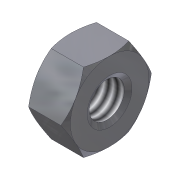
# Autodesk Inventor part: ANSI B18.2.2 - 1/4 - 20
Saved by Autodesk Inventor 2012 SP1 (Build 160190100, 190)
## iProperties
Library Location: D:\Program Files\Autodesk\Inventor 6\content
Library: local
SubLibrary: ANSI
Family: 1001
Member: 10
Member Major Revision: 1
Member Minor Revision: 2
Comments: To add or edit properties for Autodesk Inventor files, use iProperties.
Created: 2003-01-12
Part Number: ANSI B18.2.2 - 1/4 - 20
Vendor: Autodesk Inc.
Document SubType Name: Modeling
Designer: geyerm
Description: Hex Nut
Standard: ANSI B18.2.2 1/4 - 20
Material: Steel, High Strength Low Alloy
Density: 7.84 g/cm^3
Alert: To add or edit properties for Autodesk Inventor files, use iProperties.
Control State: 0
Master: False
Checked Out: False
Shininess: 64.0
Length Units: 11269
Angle Units: 11279
Time Units: 11290
Mass Units: 11283
Length Display Precision: 3
Angle Display Precision: 2
Compacted: True
EGR: 3
Classification: un/spsc 31161727
Density: 0.0
Volumn: 0.0
Area: 0.0
PropertySet Name: Model Information
Author: Autodesk
Revision Number: 2
Autodesk Inventor part; units mm, degrees
ref_plane "YZ Plane" through (0, 0, 0) normal (1, 0, 0) x (0, 1, 0)
ref_plane "XZ Plane" through (0, 0, 0) normal (0, 1, 0) x (-1, 0, 0)
ref_plane "XY Plane" through (0, 0, 0) normal (0, 0, 1) x (1, 0, 0)
sketch "Sketch1" plane through (0, 0, 0) normal (1, 0, 0) x (0, 1, 0)
  line L0 (-6.415805, 0) -> (-3.207902, 5.55625)
  line L1 (-3.207902, 5.55625) -> (3.207902, 5.55625)
  line L2 (3.207902, 5.55625) -> (6.415805, 0)
  line L3 (6.415805, 0) -> (3.207902, -5.55625)
  line L4 (3.207902, -5.55625) -> (-3.207902, -5.55625)
  line L5 (-3.207902, -5.55625) -> (-6.415805, 0)
  point P0 (0, 0)
  point P1 (0, 0)
  dimension "d0" = 12.83161
  constraints: 12 end point, 1 coincident, 1 horizontal, 11 other
  measures "d0" distance of L2.end L0.start
extrude "Body" add sketch "Sketch1" along normal blind 5.5626
sketch "Sketch2" plane through (0, 0, 0) normal (0, 0, 1) x (1, 0, 0)
  line L0 (0, 3.207902) -> (0, 6.415805)
  line L1 (0, 6.415805) -> (5.5626, 6.415805)
  line L2 (5.5626, 3.207902) -> (5.5626, 6.415805)
  line L3 (-0.55626, 0) -> (7.23138, 0)
  line L4 (0.496264, 6.415805) -> (0, 5.55625)
  line L5 (5.066336, 6.415805) -> (5.5626, 5.55625)
  dimension "d3" = 30
  dimension "d4" = 30
  dimension "d5" = 11.1125
  dimension "d6" = 11.1125
  constraints: 4 end point, 4 point on line
  measures "d3" angle of L0 L4
  measures "d4" angle of L2 L5
  measures "d5" diameter of L4.end L3
  measures "d6" diameter of L5.end L3
revolve "Chamfer1" cut sketch "Sketch2" angle 360 about axis through (-10, 0, 0) along (1, 0, 0)
sketch "Sketch3" plane through (5.5626, 0, 0) normal (1, 0, 0) x (0, 0, -1)
  arc A0 (-2.778125, -4.811854) -> (2.778125, -4.811854) centre (0, 0) ccw
  constraints: 1 coincident
hole "Thread" at (5.5626, 0, 0) direction (-1, 0, 0) diameter 4.9784 end through all thread size "1/4-20 UNC" class "2B" standard "ANSI Unified Screw Threads"
chamfer "Chamfer2" distance 0.687408 angle 30 1 edges at (5.5626, 0, 2.4892) measured on face at (5.5626, 0, 2.9892)
chamfer "Chamfer3" distance 0.687408 angle 30 1 edges at (0, 0, 2.4892) measured on face at (0, 0, 2.9892)
equation "\"d0\" = 1.1547 * SW"
equation "\"d1\" = KOH"
equation "\"d8\" = -0.5 * GD1 + 0.5 * NND"
equation "\"d40\" = -0.5 * GD1 + 0.5 * NND"
equation "\"d10\" = -0.5 * GD1 + 0.5 * NND"
equation "\"d41\" = -0.5 * GD1 + 0.5 * NND"
equation "\"d3\" = ANG1"
equation "\"d4\" = ANG2"
equation "\"d5\" = SW0"
equation "\"d6\" = SW01"
equation "\"ANG1\" = 30deg"
equation "\"ANG2\" = 30deg"
equation "\"NND\" = 6.35"
equation "\"KOH\" = 5.5626"
equation "\"SW\" = 11.1125"
equation "\"SW0\" = SW"
equation "\"SW01\" = SW"
equation "\"TOA\" = 30deg"
equation "\"THREADDIA\" = 6.35"
equation "\"E0\" = 1.155 * SW"
equation "\"GD1\" = 4.975185"
body "Solid1"
